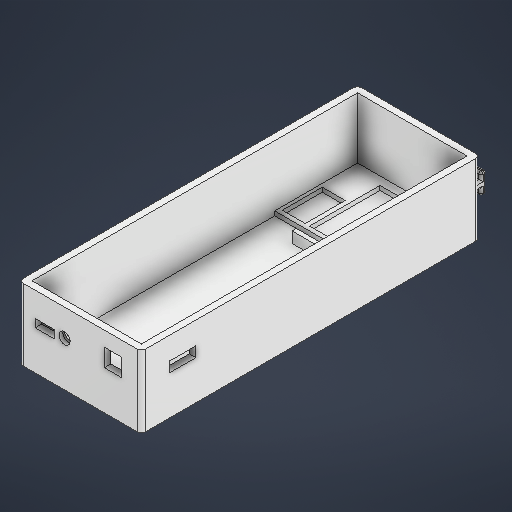
# Autodesk Inventor part: module_command
Saved by Autodesk Inventor 2025.2 (Build 292293000, 293)
## iProperties
Created: 2025-09-05
Part Number: module_command
Material: PC/ABS Plastic
Document SubType Name: Modeling
Designer: sam
Density: 1.1 g/cm^3
Appearance: Smooth - White
Author: sam
Autodesk Inventor part; units mm, degrees
ref_plane "YZ Plane" through (0, 0, 0) normal (1, 0, 0) x (0, 1, 0)
ref_plane "XZ Plane" through (0, 0, 0) normal (0, 1, 0) x (-1, 0, 0)
ref_plane "XY Plane" through (0, 0, 0) normal (0, 0, 1) x (1, 0, 0)
sketch "Sketch1" plane through (0, 0, 0) normal (0, 1, 0) x (-1, 0, 0)
  line L0 (-28.2, -78) -> (28.2, -78)
  line L1 (28.2, -78) -> (28.2, 78)
  line L2 (28.2, 78) -> (-28.2, 78)
  line L3 (-28.2, 78) -> (-28.2, -78)
  line L4 (-28.2, -78) -> (28.2, 78) construction
  line L5 (28.2, -78) -> (-28.2, 78) construction
  point P0 (0, 0)
  dimension "d0" = 56.4
  dimension "d1" = 156
  constraints: 12 end point, 2 midpoint, 2 parallel, 1 horizontal, 1 perpendicular
  measures "d0" distance of L2.end L1.end
  measures "d1" distance of L1.end L0.end
extrude "Extrusion1" add sketch "Sketch1" along normal blind 3
sketch "Sketch2" plane through (0, 3, 0) normal (0, 1, 0) x (1, 0, 0)
  line L0 (-28.2, 78) -> (-28.2, -78) projected
  line L1 (-28.2, -78) -> (28.2, -78) projected
  line L2 (28.2, -78) -> (28.2, 78) projected
  line L3 (28.2, 78) -> (-28.2, 78) projected
  line L4 (28.2, 78) -> (-28.2, 78)
  line L5 (-28.2, 78) -> (-28.2, -78)
  line L6 (-28.2, -78) -> (28.2, -78)
  line L7 (28.2, -78) -> (28.2, 78)
  line L8 (28.2, 78) -> (-28.2, -78) construction
  line L9 (-28.2, 78) -> (28.2, -78) construction
  line L10 (25.2, 75) -> (-25.2, 75)
  line L11 (-25.2, 75) -> (-25.2, -75)
  line L12 (-25.2, -75) -> (25.2, -75)
  line L13 (25.2, -75) -> (25.2, 75)
  line L14 (25.2, 75) -> (-25.2, -75) construction
  line L15 (-25.2, 75) -> (25.2, -75) construction
  point P0 (0, 0)
  dimension "d4" = 0
  dimension "d5" = 0
  dimension "d6" = 3
  dimension "d7" = 3
  constraints: 24 end point, 4 midpoint, 4 parallel, 2 horizontal, 2 perpendicular
  measures "d4" distance between parallel lines of L0 L5
  measures "d5" distance between parallel lines of L1 L6
  measures "d6" distance between parallel lines of L5 L11
  measures "d7" distance between parallel lines of L6 L12
extrude "Extrusion2" add sketch "Sketch2" along normal blind 30
fillet "Fillet1" radius 2 4 edges at (28.2, 16.5, 78) (28.2, 16.5, -78) (-28.2, 16.5, 78) (-28.2, 16.5, -78)
sketch "Sketch9" plane through (0, 3, 0) normal (0, 1, 0) x (1, 0, 0)
  line L0 (25.2, 75) -> (-25.2, 75) projected
  line L1 (-25.2, 75) -> (-25.2, -75) projected
  line L2 (-25.2, -75) -> (25.2, -75) projected
  line L3 (25.2, -75) -> (25.2, 75) projected
  line L4 (-25.2, -72.6) -> (25.2, -72.6)
  line L5 (25.2, -72.6) -> (25.2, -70.6)
  line L6 (25.2, -70.6) -> (-25.2, -70.6)
  line L7 (-25.2, -70.6) -> (-25.2, -72.6)
  line L8 (-25.2, 75) -> (-25.2, -75) projected
  line L9 (-25.2, 29.8) -> (25.2, 29.8)
  line L10 (25.2, 29.8) -> (25.2, 31.8)
  line L11 (25.2, 31.8) -> (-25.2, 31.8)
  line L12 (-25.2, 31.8) -> (-25.2, 29.8)
  line L13 (-25.2, 31.8) -> (-10.2, 31.8)
  line L14 (-10.2, 31.8) -> (-10.2, 29.8)
  line L15 (-10.2, 29.8) -> (-25.2, 29.8)
  line L16 (-25.2, 29.8) -> (-25.2, 31.8)
  point P0 (0, 0)
  point P1 (25.2, 17.2)
  point P2 (-25.2, 31.8)
  point P3 (-25.2, 29.8)
  point P4 (25.2, 29.8)
  point P5 (-25.2, -70.6)
  point P6 (25.2, -72.6)
  dimension "d79" = 2
  dimension "d80" = 2.4
  dimension "d81" = 2
  dimension "d82" = 100.4
  dimension "d87" = 15
  constraints: 24 end point, 6 parallel, 6 point on line, 3 horizontal, 3 perpendicular
  measures "d79" distance of L5.end L4.end
  measures "d80" distance between parallel lines of L2 L4
  measures "d81" distance of L10.end L9.end
  measures "d82" distance between parallel lines of L6 L9
  measures "d87" distance of L14.end L15.end
extrude "Extrusion9" add sketch "Sketch9" along normal blind 5 contours L3 L9 L14 L11 | L3 L4 L1 L6
sketch "Sketch10" plane through (0, 3, 0) normal (0, 1, 0) x (1, 0, 0)
  line L0 (-25.2, -70.6) -> (25.2, -70.6) projected
  line L1 (25.2, -70.6) -> (25.2, 29.8) projected
  line L2 (25.2, 29.8) -> (-10.2, 29.8) projected
  line L3 (-10.2, 29.8) -> (-10.2, 31.8) projected
  line L4 (-10.2, 31.8) -> (25.2, 31.8) projected
  line L5 (25.2, 31.8) -> (25.2, 75) projected
  line L6 (25.2, 75) -> (-25.2, 75) projected
  line L7 (-25.2, 75) -> (-25.2, -70.6) projected
  line L8 (-25.2, 36.8) -> (25.2, 36.8)
  line L9 (-25.2, 71.8) -> (-25.2, 36.8)
  line L10 (-25.2, 36.8) -> (25.2, 36.8)
  line L11 (25.2, 36.8) -> (25.2, 38.8)
  line L12 (25.2, 38.8) -> (-25.2, 38.8)
  line L13 (-25.2, 38.8) -> (-25.2, 36.8)
  line L14 (25.2, 31.8) -> (25.2, 75) projected
  line L15 (-25.2, 38.8) -> (25.2, 38.8)
  line L16 (25.2, 38.8) -> (25.2, 71.2)
  line L17 (25.2, 71.2) -> (-25.2, 71.2)
  line L18 (-25.2, 71.2) -> (25.2, 71.2)
  line L19 (25.2, 71.2) -> (25.2, 73.2)
  line L20 (25.2, 73.2) -> (-25.2, 73.2)
  line L21 (-25.2, 73.2) -> (-25.2, 71.2)
  line L22 (25.2, 38.8) -> (23.7, 38.8)
  line L23 (23.7, 38.8) -> (23.7, 71.2)
  line L24 (23.7, 71.2) -> (25.2, 71.2)
  line L25 (25.2, 71.2) -> (25.2, 38.8)
  line L26 (23.7, 38.8) -> (7.3, 38.8)
  line L27 (7.3, 38.8) -> (7.3, 71.2)
  line L28 (7.3, 71.2) -> (23.7, 71.2)
  line L29 (23.7, 71.2) -> (23.7, 38.8)
  line L30 (7.3, 38.8) -> (5.3, 38.8)
  line L31 (5.3, 38.8) -> (5.3, 71.2)
  line L32 (5.3, 71.2) -> (7.3, 71.2)
  line L33 (7.3, 71.2) -> (7.3, 38.8)
  line L34 (5.3, 38.8) -> (-11.1, 38.8)
  line L35 (-11.1, 38.8) -> (-11.1, 71.2)
  line L36 (-11.1, 71.2) -> (5.3, 71.2)
  line L37 (5.3, 71.2) -> (5.3, 38.8)
  line L38 (-11.1, 38.8) -> (-13.1, 38.8)
  line L39 (-13.1, 38.8) -> (-13.1, 71.2)
  line L40 (-13.1, 71.2) -> (-11.1, 71.2)
  line L41 (-11.1, 71.2) -> (-11.1, 38.8)
  line L42 (-25.2, 71.2) -> (-23.7, 71.2)
  line L43 (-23.7, 71.2) -> (-23.7, 38.8)
  line L44 (-23.7, 38.8) -> (-25.2, 38.8)
  line L45 (-25.2, 38.8) -> (-25.2, 71.2)
  line L46 (-23.7, 38.8) -> (-13.1, 38.8)
  line L47 (-13.1, 38.8) -> (-13.1, 57.2)
  line L48 (-13.1, 57.2) -> (-23.7, 57.2)
  line L49 (-23.7, 57.2) -> (-23.7, 38.8)
  point P0 (0, 0)
  point P1 (25.2, 73.2)
  point P2 (-25.2, 73.2)
  point P3 (25.2, 36.8)
  point P4 (5.3, 38.8)
  point P5 (-13.1, 38.8)
  point P6 (-23.7, 38.8)
  point P7 (-23.7, 57.2)
  point P8 (23.7, 38.8)
  point P9 (7.3, 38.8)
  dimension "d89" = 5
  dimension "d90" = 2
  dimension "d91" = 32.4
  dimension "d92" = 2
  dimension "d93" = 1.5
  dimension "d94" = 16.4
  dimension "d95" = 2
  dimension "d96" = 16.4
  dimension "d97" = 2
  dimension "d98" = 1.5
  dimension "d99" = 18.4
  constraints: 82 end point, 19 parallel, 11 horizontal, 10 perpendicular, 10 point on line
  measures "d89" distance between parallel lines of L4 L8
  measures "d90" distance of L11.end L10.end
  measures "d91" distance of L16.end L15.end
  measures "d92" distance of L19.end L18.end
  measures "d93" distance of L23.end L24.end
  measures "d94" distance of L27.end L28.end
  measures "d95" distance of L31.end L32.end
  measures "d96" distance of L35.end L36.end
  measures "d97" distance of L39.end L40.end
  measures "d98" distance of L43.end L44.end
  measures "d99" distance of L47.end L46.end
extrude "Extrusion10" add sketch "Sketch10" along normal blind 2 contours L7 L12 L5 L8 | L7 L17 L43 L12 | L7 L20 L5 L17 | L12 L23 L17 L5 | L17 L39 L48 L43 | L39 L17 L35 L12 | L7 L6 L5 L20 | L12 L31 L17 L27
sketch "Sketch11" plane through (-23.2, 5, 78) normal (0, 0, 1) x (1, 0, 0)
  line L0 (-3, 28) -> (49.4, 28) projected
  line L1 (2.5, 13) -> (11.2, 13)
  line L2 (11.2, 13) -> (11.2, 16.7)
  line L3 (11.2, 16.7) -> (2.5, 16.7)
  line L4 (2.5, 16.7) -> (2.5, 13)
  line L5 (42.4, 13) -> (34.34, 13)
  line L6 (34.34, 13) -> (34.34, 21.2)
  line L7 (34.34, 21.2) -> (42.4, 21.2)
  line L8 (42.4, 21.2) -> (42.4, 13)
  circle A0 centre (16, 15.6) radius 2.6
  line L9 (48.4, 0) -> (48.4, 30) projected
  line L10 (49.4, 28) -> (49.4, -5) projected
  line L11 (-3, -5) -> (-3, 28) projected
  line L12 (-3, -5) -> (49.4, -5) projected
  line L13 (51.4, -5) -> (51.4, 28) projected
  line L14 (-5, 28) -> (-5, -5) projected
  point P0 (23.2, -5)
  point P1 (46.4, 0)
  point P2 (0, 0)
  dimension "d110" = 8.7
  dimension "d111" = 3.7
  dimension "d112" = 8.06
  dimension "d113" = 8.2
  dimension "d114" = 5.2
  dimension "d149" = 9
  dimension "d150" = 7.5
  dimension "d151" = 21
  dimension "d152" = 18
  dimension "d153" = 18
  dimension "d154" = 18
  constraints: 16 end point, 4 parallel, 2 horizontal, 2 perpendicular, 1 centre point
  measures "d110" distance of L3.end L2.end
  measures "d111" distance of L2.end L1.end
  measures "d112" distance of L6.end L7.end
  measures "d113" distance of L5.end L6.end
  measures "d114" diameter of A0
  measures "d149" distance between parallel lines of L8 L13
  measures "d150" distance between parallel lines of L14 L4
  measures "d151" distance from line of A0.centre L14
  measures "d152" distance between parallel lines of L12 L5
  measures "d153" distance between parallel lines of L12 L1
  measures "d154" distance edge to line of A0 L12
extrude "Extrusion11" cut sketch "Sketch11" against normal blind 3 contours L4 L3 L2 L1 | L5 L6 L7 L8 | A0
sketch "Sketch12" plane through (25.2, 3, 75) normal (0, 0, -1) x (-1, 0, 0)
  line L0 (14.06, 23.2) -> (14.06, 15) projected
  line L1 (14.06, 15) -> (6, 15) projected
  line L2 (6, 15) -> (6, 23.2) projected
  line L3 (6, 23.2) -> (14.06, 23.2) projected
  line L4 (37.2, 18.7) -> (45.9, 18.7) projected
  line L5 (45.9, 18.7) -> (45.9, 15) projected
  line L6 (45.9, 15) -> (37.2, 15) projected
  line L7 (37.2, 15) -> (37.2, 18.7) projected
  circle A0 centre (32.4, 17.6) radius 2.6 projected
  line L8 (50.4, 0) -> (0, 0) projected
  line L9 (50.4, 0) -> (50.4, 30) projected
  line L10 (0, 30) -> (50.4, 30) projected
  line L11 (0, 0) -> (0, 30) projected
  circle A1 centre (32.4, 17.6) radius 3.05
  point P0 (25.2, -3)
  dimension "d128" = 6.1
  constraints: 1 centre point, 1 coincident
  measures "d128" diameter of A1
extrude "Extrusion12" cut sketch "Sketch12" against normal blind 1.2 contours A1
sketch "Sketch13" plane through (23.2, 5, -78) normal (0, 0, -1) x (-1, 0, 0)
  line L0 (-2, 18) -> (48.4, 18)
  line L1 (48.4, 18) -> (48.4, 8.4)
  line L2 (48.4, 8.4) -> (-2, 8.4)
  line L3 (-2, 8.4) -> (-2, 18)
  line L4 (51.4, -5) -> (51.4, 28) projected
  line L5 (-5, 28) -> (-5, -5) projected
  line L6 (-3, -5) -> (49.4, -5) projected
  point P0 (23.2, -5)
  point P1 (51.4, 0)
  point P2 (-5, 0)
  point P3 (51.4, 11.5)
  point P4 (48.4, 13.2)
  dimension "d131" = 9.6
  dimension "d146" = 3
  dimension "d147" = 3
  dimension "d156" = 23
  constraints: 8 end point, 2 midpoint, 2 parallel, 1 horizontal, 1 perpendicular
  measures "d131" distance of L0.end L1.end
  measures "d146" distance between parallel lines of L1 L4
  measures "d147" distance between parallel lines of L5 L3
  measures "d156" distance between parallel lines of L0 L6
extrude "Extrusion13" add sketch "Sketch13" along normal blind 6
sketch "Sketch14" plane through (-25.2, 13.4, -78) normal (-1, 0, 0) x (0, 0, 1)
  line L0 (0, 9.6) -> (0, 0) projected
  line L1 (0, 9.6) -> (-6, 9.6) projected
  line L2 (-6, 0) -> (-6, 9.6) projected
  line L3 (0, 0) -> (-6, 0) projected
  line L4 (0, 9.6) -> (-3.4, 9.6)
  line L5 (-3.4, 9.6) -> (-3.4, 6.6)
  line L6 (-3.4, 6.6) -> (0, 6.6)
  line L7 (0, 6.6) -> (0, 9.6)
  line L8 (0, 0) -> (-3.4, 0)
  line L9 (-3.4, 0) -> (-3.4, 3)
  line L10 (-3.4, 3) -> (0, 3)
  line L11 (0, 3) -> (0, 0)
  point P0 (78, -13.4)
  point P1 (0, 6.6)
  dimension "d137" = 3.4
  dimension "d138" = 3
  dimension "d139" = 3.4
  dimension "d140" = 3
  constraints: 16 end point, 4 parallel, 2 horizontal, 2 perpendicular
  measures "d137" distance of L6.end L5.end
  measures "d138" distance of L5.end L4.end
  measures "d139" distance of L9.end L10.end
  measures "d140" distance of L8.end L9.end
extrude "Extrusion14" cut sketch "Sketch14" against normal up to surface (50.4 mm away) contours L0 L6 L5 L1 | L0 L3 L9 L10
fillet "Fillet5" radius 1 18 edges at (0, 23, -84) (0, 23, -81.4) (0, 13.4, -84) (0, 13.4, -81.4) (-25.2, 16.4, -79.7) (-25.2, 20, -79.7) (25.2, 16.4, -79.7) (25.2, 20, -79.7) (-25.2, 18.2, -84) (-25.2, 21.5, -81.4) (-25.2, 14.9, -81.4) (-25.2, 23, -82.7) (-25.2, 13.4, -82.7) (25.2, 23, -82.7) (25.2, 13.4, -82.7) (25.2, 14.9, -81.4) (25.2, 18.2, -84) (25.2, 21.5, -81.4)
sketch "Sketch15" plane through (28.2, 0, 76) normal (1, 0, 0) x (0, 0, -1)
  line L0 (11, 22.7) -> (23.1, 22.7)
  line L1 (23.1, 22.7) -> (23.1, 18)
  line L2 (23.1, 18) -> (11, 18)
  line L3 (11, 18) -> (11, 22.7)
  line L4 (-2, 33) -> (-2, 0) projected
  line L5 (0, 0) -> (152, 0) projected
  point P0 (76, 0)
  dimension "d157" = 12.1
  dimension "d158" = 4.7
  dimension "d159" = 13
  dimension "d160" = 18
  constraints: 8 end point, 2 parallel, 1 horizontal, 1 perpendicular
  measures "d157" distance of L1.end L2.end
  measures "d158" distance of L0.end L1.end
  measures "d159" distance between parallel lines of L4 L3
  measures "d160" distance between parallel lines of L5 L2
extrude "Extrusion15" cut sketch "Sketch15" against normal blind 3
body "Solid1"
